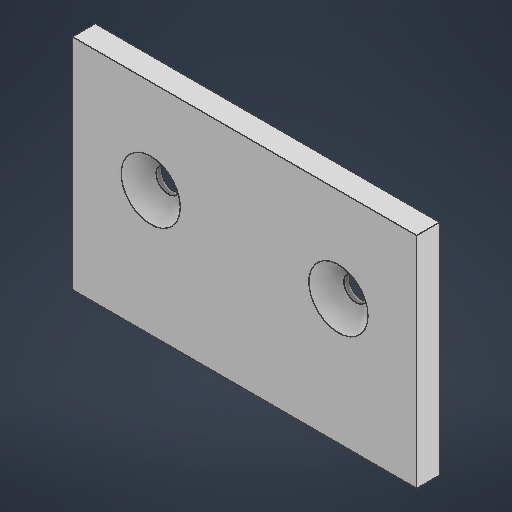
# Autodesk Inventor part: plaka
Saved by Autodesk Inventor 2025.4 (Build 294407000, 407)
## iProperties
Created: 2026-06-20
Part Number: plaka
Material: Generic
Document SubType Name: Modeling
Designer: yigithan
Density: 1 g/cm^3
Appearance: Default
Author: yigithan
Autodesk Inventor part; units mm, degrees
ref_plane "YZ Plane" through (0, 0, 0) normal (1, 0, 0) x (0, 1, 0)
ref_plane "XZ Plane" through (0, 0, 0) normal (0, 1, 0) x (-1, 0, 0)
ref_plane "XY Plane" through (0, 0, 0) normal (0, 0, 1) x (1, 0, 0)
sketch "Sketch1" plane through (0, 0, 0) normal (0, 0, 1) x (1, 0, 0)
  line L0 (-34.925, -22.225) -> (34.925, -22.225)
  line L1 (34.925, -22.225) -> (34.925, 22.225)
  line L2 (34.925, 22.225) -> (-34.925, 22.225)
  line L3 (-34.925, 22.225) -> (-34.925, -22.225)
  line L4 (-34.925, -22.225) -> (34.925, 22.225) construction
  line L5 (34.925, -22.225) -> (-34.925, 22.225) construction
  point P0 (0, 0)
  dimension "d0" = 69.85
  dimension "d1" = 44.45
  constraints: 12 end point, 2 midpoint, 2 parallel, 1 horizontal, 1 perpendicular
  measures "d0" distance of L2.end L1.end
  measures "d1" distance of L1.end L0.end
extrude "Extrusion1" add sketch "Sketch1" along normal blind 4.64
sketch "Sketch2" plane through (0, 0, 4.64) normal (0, 0, 1) x (1, 0, 0)
  line L0 (-34.925, -22.225) -> (34.925, -22.225) projected
  line L1 (-34.925, 22.225) -> (-34.925, -22.225) projected
  point P0 (0, 0)
  point P1 (-19.045, 3.175)
  point P2 (19.055, 3.175)
  dimension "d4" = 25.4
  dimension "d5" = 15.88
  dimension "d6" = 38.1
  constraints: 1 horizontal alignment
  measures "d4" distance from line of L0 point (-19.045, 3.175)
  measures "d5" distance from line of L1 point (-19.045, 3.175)
  measures "d6" distance of point (19.055, 3.175) point (-19.045, 3.175)
hole "Hole1" at (-19.045, 3.175, 4.64) at (19.055, 3.175, 4.64) direction (0, 0, -1) diameter 4.917 depth 15 tip angle 118 countersink diameter 12 countersink angle 90 thread size "M6x1" class "6H" standard "ANSI Metric M Profile"
body "Solid1"
